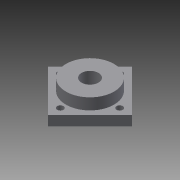
# Autodesk Inventor part: ff12
Saved by Autodesk Inventor 2014 (Build 180170000, 170)
## iProperties
Created: 2014-08-22
Part Number: ff12
Material: Generic
Document SubType Name: Modeling
Designer: Matthew
Density: 1 g/cm^3
Appearance: Default
Author: Matthew
Autodesk Inventor part; units mm, degrees
ref_plane "YZ Plane" through (0, 0, 0) normal (1, 0, 0) x (0, 1, 0)
ref_plane "XZ Plane" through (0, 0, 0) normal (0, 1, 0) x (-1, 0, 0)
ref_plane "XY Plane" through (0, 0, 0) normal (0, 0, 1) x (1, 0, 0)
sketch "Sketch1" plane through (0, 0, 0) normal (0, 0, 1) x (1, 0, 0)
  circle A0 centre (0, 0) radius 17 construction
  circle A1 centre (0, 0) radius 6 construction
  line L0 (-29.6985, 0) -> (0, 29.6985)
  line L1 (0, 29.6985) -> (29.6985, 0)
  line L2 (29.6985, 0) -> (0, -29.6985)
  line L3 (0, -29.6985) -> (-29.6985, 0)
  line L4 (-29.6985, 0) -> (29.6985, 0) construction
  line L5 (0, 29.6985) -> (0, -29.6985) construction
  point P0 (0, 21)
  point P1 (21, 0)
  point P2 (-21, 0)
  point P3 (0, -21)
  dimension "d0" = 34
  dimension "d1" = 12
  dimension "d2" = 21
  dimension "d3" = 21
  dimension "d4" = 21
  dimension "d5" = 21
  dimension "d6" = 21
  dimension "d7" = 42
  dimension "d8" = 42
  constraints: 12 end point, 2 centre point, 2 coincident, 2 horizontal alignment, 2 midpoint, 2 parallel, 1 horizontal, 1 perpendicular, 1 vertical alignment
  measures "d0" diameter of A0
  measures "d1" diameter of A1
  measures "d2" horizontal distance of point (21, 0) point (0, -21)
  measures "d3" horizontal distance of point (0, -21) point (21, 0)
  measures "d4" horizontal distance of point (-21, 0) point (0, 21)
  measures "d5" horizontal distance of point (-21, 0) point (0, -21)
  measures "d6" distance of point (0, 0) point (21, 0)
  measures "d7" distance of L0.start L0.end
  measures "d8" distance of L0.end L1.end
extrude "Extrusion1" add sketch "Sketch1" along normal blind 7
sketch "Sketch2" plane through (0, 0, 7) normal (0, 0, 1) x (1, 0, 0)
  circle A0 centre (0, 0) radius 6
  circle A1 centre (0, 0) radius 18
  circle A2 centre (0, 21) radius 2.25
  circle A3 centre (21, 0) radius 2.25
  circle A4 centre (0, -21) radius 2.25
  circle A5 centre (-21, 0) radius 2.25
  dimension "d11" = 12
  dimension "d12" = 36
  dimension "d13" = 4.5
  dimension "d14" = 4.5
  dimension "d15" = 4.5
  dimension "d16" = 4.5
  dimension "d17" = 21
  dimension "d18" = 21
  dimension "d19" = 21
  dimension "d20" = 21
  constraints: 6 centre point, 2 coincident, 2 horizontal alignment, 2 vertical alignment
  measures "d11" diameter of A0
  measures "d12" diameter of A1
  measures "d13" diameter of A2
  measures "d14" diameter of A3
  measures "d15" diameter of A4
  measures "d16" diameter of A5
  measures "d17" horizontal distance of A2.centre A3.centre
  measures "d18" horizontal distance of A3.centre A2.centre
  measures "d19" horizontal distance of A5.centre A4.centre
  measures "d20" distance of point (0, 0) A5.centre
extrude "Extrusion2" cut sketch "Sketch2" against normal blind 20 contours A2 | A3 | A4 | A5
sketch "Sketch3" plane through (0, 0, 7) normal (0, 0, 1) x (1, 0, 0)
  circle A0 centre (0, 0) radius 17
  circle A1 centre (0, 0) radius 6
  dimension "d23" = 34
  dimension "d24" = 12
  constraints: 2 centre point, 2 coincident
  measures "d23" diameter of A0
  measures "d24" diameter of A1
extrude "Extrusion3" cut sketch "Sketch3" against normal blind 20 contours A1
sketch "Sketch4" plane through (0, 0, 7) normal (0, 0, 1) x (1, 0, 0)
  circle A0 centre (0, 0) radius 6 projected
  circle A1 centre (0, 0) radius 17
  dimension "d27" = 34
  constraints: 1 centre point, 1 coincident
  measures "d27" diameter of A1
extrude "Extrusion4" add sketch "Sketch4" along normal blind 8
chamfer "Chamfer1" distance 4 angle 45 1 edges at (0, 29.6985, 3.5)
chamfer "Chamfer2" distance 4 angle 45 1 edges at (29.6985, 0, 3.5)
chamfer "Chamfer3" distance 4 angle 45 1 edges at (-29.6985, 0, 3.5)
chamfer "Chamfer4" distance 4 angle 45 1 edges at (0, -29.6985, 3.5)
equation "\"d2\" = d3"
equation "\"d4\" = d3"
equation "\"d5\" = d3"
equation "\"d14\" = d13"
equation "\"d15\" = d13"
equation "\"d16\" = d13"
equation "\"d18\" = d17"
equation "\"d19\" = d17"
equation "\"d20\" = d17"
body "Solid1"
